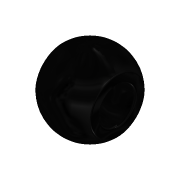
# Autodesk Inventor part: RBPB5ball
Saved by Autodesk Inventor 2021 (Build 250183000, 183)
## iProperties
Part Number: RBPB5ball
Material: Allgemein
Catalog Web Link: www.cadenas.de
Description: RBPB_ball-Spherical Bearings - Standard Type
Vendor: MISUMI
Document SubType Name: Modeling
Designer: partserver
Manufacturer: MISUMI
Mass: 0.48399 g
Surface Area: 4.54513 cm^2
Volume: 0.48399 cm^3
Density: 1 g/cm^3
Appearance: Schwarz
Category: PARTsolutions
Company: MISUMI
PSOL_IDENT_0: {$CADENAS_DATA\23d-libs\misumi\metric\34_cylinders\rbpb_ball.prj},161 {VTYP=3D},{NB=RBPB5ball},{LINA=
PSOL_IDENT_1: RBPB5ball},{NN=RBPB_ball},{DATE=30.06.2021 13:14:18},{GEOMDATE=11.07.2011 00:00:00},{VERSION=},{LINE
PSOL_IDENT_2: ID=10},{WBVAR=},{WBNUMERIC=}  {NB=RBPB5ball},{LINA=RBPB5ball},{KT=DUMMY},{PN=RBPB5},{TYPE=RBPB},{MAT
PSOL_IDENT_3: H=1035 Steel},{MATSIR=51200 Bearing Steel},{STSIR=Hard Chrome Plating},{HARDSIR=58HRC~},{MATB=Specia
PSOL_IDENT_4: l Copper Alloy},{DD=5},{D=16},{B=6.00},{B1=8},{DD1=7.7},{H=1.0},{R=0.3},{BD=11.112},{A1=8},{A11=8},{
PSOL_IDENT_5: A2=13},{A3=30},{SLC=7.84},{SLC1=7.84},{MASS=8.5},{RDC=0.035mm or Less},{ADC=0.1mm or Less}
NB: RBPB5ball
NN: RBPB_ball
NT: Spherical Bearings - Standard Type
NBSYN: $PN.ball
LINA: RBPB5ball
CATALOG: Misumi
MATSIR: 51200 Bearing Steel
DD: 5
D: 16
B: 6
B1: 8
DD1: 7.7
H: 1
R: 0.3
BD: 11.112
A11: 8
A2: 13
A3: 30
SLC1: 7.84
MASS: 8.5
ADC: 0.1mm or Less
SUPPLIER: MISUMI
ARTICLENO: RBPB5ball
BOMINFO: RBPB5ball
CREATOR: CADENAS GmbH
Title: RBPB5ball
Author: Cadenas PARTsolutions
Comments: Spherical Bearings - Standard Type
Autodesk Inventor part; units mm, degrees
sketch "Sketch_1" plane through (0, 0, 0) normal (0, 0, 1) x (1, 0, 0)
  line L0 (4, 0) -> (-4, 0)
  arc A0 (-4, 2.8) -> (-3.7, 2.5) centre (-3.7, 2.8) ccw
  line L1 (-3.7, 2.5) -> (3.7, 2.5)
  arc A1 (3.7, 2.5) -> (4, 2.8) centre (3.7, 2.8) ccw
  line L2 (4, 2.8) -> (4, 3.733)
  arc A2 (4, 3.733) -> (3.9112, 3.9461) centre (3.7, 3.733) ccw
  arc A3 (3.9112, 3.9461) -> (-3.9112, 3.9461) centre (0, 0) ccw
  arc A4 (-3.9112, 3.9461) -> (-4, 3.733) centre (-3.7, 3.733) ccw
  line L3 (-4, 3.733) -> (-4, 2.8)
  constraints: 10 point on circle, 8 end point, 5 centre point
revolve "Revolution1" add sketch "Sketch_1" angle 360 about axis through (4, 0, 0) along (1, 0, 0)
ref_plane "ball_XY" through (0, 0, 0) normal (1, 0, 0) x (0, 0, -1)
ref_plane "ball_YZ" through (0, 0, 0) normal (0, 0, -1) x (0, 1, 0)
ref_plane "ball_ZX" through (0, 0, 0) normal (0, 1, 0) x (1, 0, 0)
body "Solid1"
